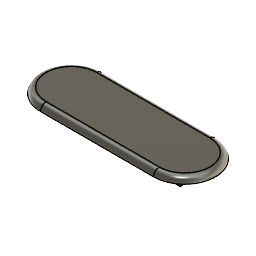
Canal - top plate v12 (Autodesk Fusion 360 design; units mm, degrees)
Autodesk Fusion 360 part; units mm, degrees
sketch "Sketch1" plane through (0, 0, 0) normal (0, 0, 1) x (1, 0, 0)
  line L0 (82.0141, 54.0159) -> (121.4141, 54.0159)
  line L1 (121.4141, 32.4159) -> (82.0141, 32.4159)
  arc A0 (82.0141, 54.0159) -> (71.257, 42.2547) centre (82.0141, 43.2159) ccw
  arc A1 (71.257, 42.2547) -> (82.0141, 32.4159) centre (82.0141, 43.2159) ccw
  arc A2 (130.5847, 37.5114) -> (121.4141, 54.0159) centre (121.4141, 43.2159) ccw
  arc A3 (121.4141, 32.4159) -> (130.5847, 37.5114) centre (121.4141, 43.2159) ccw
  dimension "d1" = 21.6
  dimension "d58" = 39.4
  constraint horizontal L0
  constraint horizontal L1
  constraint tangent L0 A0
  constraint tangent L1 A1
  constraint coincident A0.end A1.start
  constraint tangent L0 A2
  constraint tangent L1 A3
  constraint coincident A2.start A3.end
  constraint coincident A2.centre A3.centre
  constraint coincident A0.centre A1.centre
  measures "d1" distance of L0 L1
  measures "d58" distance of A0.centre A2.centre
extrude "Extrude1" add sketch "Sketch1" along normal blind 2
fillet "Fillet1" radius 2 4 edges at (132.2141, 43.2159, 2) (101.7141, 54.0159, 2) (71.2141, 43.2159, 2) (101.7141, 32.4159, 2)
sketch "Sketch4" plane through (0, 0, 0) normal (0, 0, -1) x (1, 0, 0)
  arc A0 (82.0141, -32.4159) -> (82.0141, -54.0159) centre (82.0141, -43.2159) ccw
  line L0 (82.0141, -54.0159) -> (121.4141, -54.0159)
  arc A1 (121.4141, -54.0159) -> (121.4141, -32.4159) centre (121.4141, -43.2159) ccw
  line L1 (121.4141, -32.4159) -> (82.0141, -32.4159)
  line L2 (71.2141, -43.2159) -> (132.2141, -43.2159) construction
  line L3 (88.4141, -37.1159) -> (88.4141, -49.3159)
  line L4 (101.7141, -32.4159) -> (101.7141, -54.0159) construction
  line L5 (72.4941, -38.1159) -> (87.4141, -38.1159)
  line L6 (87.4141, -38.1159) -> (87.4141, -48.3159)
  line L7 (87.4141, -48.3159) -> (72.4941, -48.3159)
  line L8 (77.4372, -37.1159) -> (88.4141, -37.1159)
  line L9 (88.4141, -49.3159) -> (77.4372, -49.3159)
  line L10 (77.4372, -37.1159) -> (77.4372, -49.3159)
  line L11 (115.0141, -49.3159) -> (125.991, -49.3159)
  line L12 (116.0141, -48.3159) -> (130.9341, -48.3159)
  line L13 (125.991, -37.1159) -> (125.991, -49.3159)
  line L14 (130.9341, -38.1159) -> (116.0141, -38.1159)
  line L15 (125.991, -37.1159) -> (115.0141, -37.1159)
  line L16 (116.0141, -38.1159) -> (116.0141, -48.3159)
  line L17 (115.0141, -37.1159) -> (115.0141, -49.3159)
  dimension "d18" = 17.2
  dimension "d20" = 1
  dimension "d35" = 1
  dimension "d51" = 12.2
  dimension "d52" = 1
  constraint midpoint A0 L2.start
  constraint midpoint A1 L2.end
  constraint vertical L3
  constraint midpoint L1 L4.start
  constraint midpoint L0 L4.end
  constraint coincident A0 L5.start
  constraint horizontal L5
  constraint perpendicular L5 L6
  constraint coincident A0 L7.end
  constraint perpendicular L6 L7
  constraint symmetric L2 L5 L7
  constraint perpendicular L3 L8
  constraint perpendicular L3 L9
  constraint vertical L10
  constraint coincident L9.end L10.end
  constraint symmetric L3.start L4 L15.end
  constraint symmetric L3.end L4 L11.start
  constraint symmetric L4 L5.start L14.start
  constraint symmetric L4 L5.end L14.end
  constraint symmetric L4 L6.end L12.start
  constraint symmetric L4 L7.end L12.end
  constraint symmetric L4 L8.start L13.start
  constraint symmetric L4 L9.end L11.end
  measures "d18" distance of L2.start L3
  measures "d20" distance of L3 L6
  measures "d35" distance of L5 L8
  measures "d51" distance of L3.start L3.end
  measures "d52" distance of L7 L9
extrude "Extrude3" add sketch "Sketch4" along normal blind 3 contours L3 L5 L6 L7 L8 L9 L10 | L11 L12 L13 L14 L15 L16 L17
sketch "Sketch6" plane through (87.4141, 0, 0) normal (-1, 0, 0) x (0, -1, 0)
  line L0 (-38.1159, 0) -> (-48.3159, 0)
  line L1 (-48.3159, 0) -> (-48.3159, -3)
  line L2 (-48.3159, -3) -> (-38.1159, -3)
  line L3 (-38.1159, -3) -> (-38.1159, 0)
  line L4 (-43.2159, -3) -> (-43.2159, 0) construction
  line L5 (-42.1159, -2.4) -> (-44.3159, -2.4)
  line L6 (-44.3159, -2.4) -> (-44.3159, -1.2)
  line L7 (-44.3159, -1.2) -> (-42.1159, -1.2)
  line L8 (-42.1159, -1.2) -> (-42.1159, -2.4)
  dimension "d23" = 2.2
  dimension "d24" = 1.2
  dimension "d25" = 0.6
  constraint midpoint L2 L4.start
  constraint midpoint L0 L4.end
  constraint horizontal L5
  constraint vertical L6
  constraint horizontal L7
  constraint vertical L8
  constraint symmetric L4 L6 L8
  measures "d23" distance of L5.start L5.end
  measures "d24" distance of L5.end L6.end
  measures "d25" distance of L2 L5
extrude "Extrude4" cut sketch "Sketch6" against normal blind 33 contours L5 L6 L7 L8
